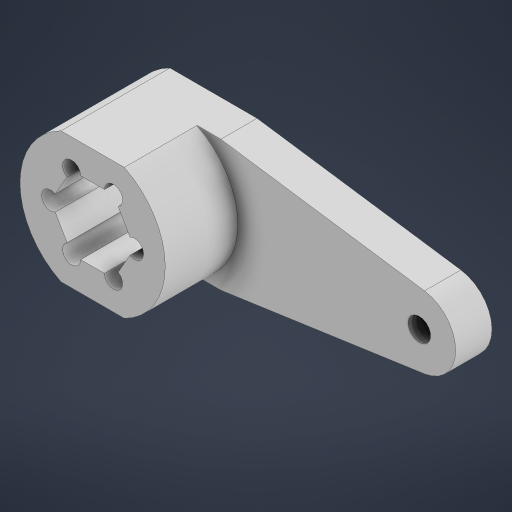
# Autodesk Inventor part: Lower Linkage
Saved by Autodesk Inventor 2023 (Build 270158000, 158)
## iProperties
Created: 2022-05-02
Part Number: Lower Linkage
Material: Generic
Document SubType Name: Modeling
Designer: FizzyApple12
Density: 1 g/cm^3
Appearance: Default
Author: FizzyApple12
Autodesk Inventor part; units mm, degrees
ref_plane "YZ Plane" through (0, 0, 0) normal (1, 0, 0) x (0, 1, 0)
sketch "Sketch1" plane through (0, 0, 0) normal (0, 0, 1) x (1, 0, 0)
  line L0 (7.3323, 0) -> (3.6662, -6.35)
  line L1 (3.6662, -6.35) -> (-3.6662, -6.35)
  line L2 (-3.6662, -6.35) -> (-7.3323, 0)
  line L3 (-7.3323, 0) -> (-3.6662, 6.35)
  line L4 (-3.6662, 6.35) -> (3.6662, 6.35)
  line L5 (3.6662, 6.35) -> (7.3323, 0)
  circle A0 centre (0, 0) radius 12.7
  circle A1 centre (44.45, 0) radius 6.35
  line L6 (45.3571, 6.2849) -> (1.8143, 12.5697)
  line L7 (45.3571, -6.2849) -> (1.8143, -12.5697)
  line L8 (0, 0) -> (64.5311, 0) construction
  dimension "d0" = 12.7
  dimension "d1" = 25.4
  dimension "d2" = 44.45
  dimension "d3" = 12.7
  constraints: 18 end point, 9 coincident, 4 point on circle, 4 tangent, 2 centre point, 1 horizontal, 1 parallel, 1 point on line, 13 other
  measures "d0" distance between parallel lines of L1 L4
  measures "d1" diameter of A0
  measures "d2" distance of point (0, 0) point (44.45, 0)
  measures "d3" diameter of A1
extrude "Extrusion1" add sketch "Sketch1" along normal blind 6.35
hole "Hole1" at (44.45, 0, 0) direction (0, 0, 1) diameter 3.9624 depth 13.6144 thread size "10-32 UNF" class "2B" standard "ANSI Unified Screw Threads"
hole "Hole2" at (3.6662, -6.35, 0) at (7.3323, 0, 0) at (3.6662, 6.35, 0) at (-3.6662, 6.35, 0) at (-7.3323, 0, 0) at (-3.6662, -6.35, 0) direction (0, 0, 1) diameter 3.175 depth 13.6144
sketch "Sketch2" plane through (0, 0, 6.35) normal (0, 0, 1) x (1, 0, 0)
  arc A0 (1.8143, 12.5697) -> (1.8143, -12.5697) centre (0, 0) ccw projected
  circle A1 centre (0, 0) radius 12.7
  line L0 (-2.0787, 6.35) -> (2.0787, 6.35) projected
  arc A2 (4.4599, 4.9752) -> (2.0787, 6.35) centre (3.6662, 6.35) ccw projected
  arc A3 (-2.0787, 6.35) -> (-4.4599, 4.9752) centre (-3.6662, 6.35) ccw projected
  line L1 (-6.5386, 1.3748) -> (-4.4599, 4.9752) projected
  arc A4 (-6.5386, 1.3748) -> (-6.5386, -1.3748) centre (-7.3323, 0) ccw projected
  line L2 (-4.4599, -4.9752) -> (-6.5386, -1.3748) projected
  arc A5 (-4.4599, -4.9752) -> (-2.0787, -6.35) centre (-3.6662, -6.35) ccw projected
  line L3 (2.0787, -6.35) -> (-2.0787, -6.35) projected
  arc A6 (2.0787, -6.35) -> (4.4599, -4.9752) centre (3.6662, -6.35) ccw projected
  line L4 (6.5386, -1.3748) -> (4.4599, -4.9752) projected
  arc A7 (6.5386, -1.3748) -> (6.5386, 1.3748) centre (7.3323, 0) ccw projected
  line L5 (4.4599, 4.9752) -> (6.5386, 1.3748) projected
  point P0 (1.8143, -12.5697)
  constraints: 1 coincident, 3 other
extrude "Extrusion2" add sketch "Sketch2" along normal blind 12.7
chamfer "Chamfer1" [suppressed]
ref_plane "Work Plane1" through (-2.0787, -11.43, 0) normal (0, 1, 0) x (1, 0, 0)
sketch "Sketch3" plane through (-2.0787, -11.43, 0) normal (0, 1, 0) x (1, 0, 0)
  line L0 (-10.6213, 0) -> (3.893, 0) projected
  line L1 (-10.6213, -19.05) -> (14.7787, -19.05) projected
  line L2 (-10.6213, 0) -> (14.7787, 0)
  line L3 (14.7787, 0) -> (14.7787, -19.05)
  line L4 (14.7787, -19.05) -> (-10.6213, -19.05)
  line L5 (-10.6213, -19.05) -> (-10.6213, 0)
  point P0 (2.0787, 0)
  point P1 (-10.6213, -19.05)
  constraints: 8 end point, 2 parallel, 1 horizontal, 1 perpendicular
extrude "Extrusion3" cut sketch "Sketch3" against normal through all
ref_plane "Work Plane2" through (-2.0787, 11.43, 0) normal (0, -1, 0) x (1, 0, 0)
sketch "Sketch4" plane through (-2.0787, 11.43, 0) normal (0, -1, 0) x (1, 0, 0)
  line L0 (3.893, 0) -> (-10.6213, 0) projected
  line L1 (14.7787, 19.05) -> (-10.6213, 19.05) projected
  line L2 (-10.6213, 0) -> (14.7787, 0)
  line L3 (14.7787, 0) -> (14.7787, 19.05)
  line L4 (14.7787, 19.05) -> (-10.6213, 19.05)
  line L5 (-10.6213, 19.05) -> (-10.6213, 0)
  point P0 (2.0787, 0)
  point P1 (-3.4571, 0)
  point P2 (7.6145, 19.05)
  point P3 (-3.4571, 19.05)
  point P4 (-10.6213, 19.05)
  constraints: 8 end point, 2 parallel, 1 horizontal, 1 perpendicular
extrude "Extrusion4" cut sketch "Sketch4" against normal through all
body "Solid1"
